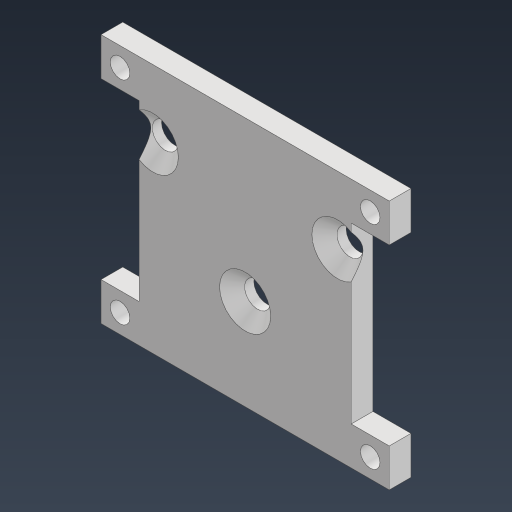
# Autodesk Inventor part: vesc_holder
Saved by Autodesk Inventor 2023 (Build 270158000, 158)
## iProperties
Created: 2026-01-23
Part Number: vesc_holder
Material: Generic
Document SubType Name: Modeling
Designer: szymo
Density: 1 g/cm^3
Appearance: Default
Author: szymo
Autodesk Inventor part; units mm, degrees
ref_plane "YZ Plane" through (0, 0, 0) normal (1, 0, 0) x (0, 1, 0)
ref_plane "XZ Plane" through (0, 0, 0) normal (0, 1, 0) x (-1, 0, 0)
ref_plane "XY Plane" through (0, 0, 0) normal (0, 0, 1) x (1, 0, 0)
sketch "Sketch1" plane through (0, 0, 0) normal (0, 0, 1) x (1, 0, 0)
  circle A0 centre (16.975, 77.075) radius 1.621 projected
  circle A1 centre (0, 60.25) radius 1.621 projected
  circle A2 centre (-16.975, 77.075) radius 1.621 projected
  line L0 (-19.5, 89.5) -> (-19.5, 43.5) projected
  line L1 (-19.5, 43.5) -> (-13.8, 43.5) projected
  line L2 (-13.8, 43.5) -> (-13.8, 49.1) projected
  arc A3 (-10.8, 52.1) -> (-13.8, 49.1) centre (-10.8, 49.1) ccw projected
  line L3 (-10.8, 52.1) -> (10.8, 52.1) projected
  arc A4 (13.8, 49.1) -> (10.8, 52.1) centre (10.8, 49.1) ccw projected
  line L4 (13.8, 49.1) -> (13.8, 43.5) projected
  line L5 (13.8, 43.5) -> (19.5, 43.5) projected
  line L6 (19.5, 43.5) -> (19.5, 89.5) projected
  line L7 (19.5, 89.5) -> (-19.5, 89.5) projected
  circle A5 centre (-17, 46.5) radius 1.25 projected
  circle A6 centre (17, 46.5) radius 1.25 projected
  circle A7 centre (17, 86.5) radius 1.25 projected
  circle A8 centre (-17, 86.5) radius 1.25 projected
  line L8 (-19.5, 89.5) -> (19.5, 89.5)
  line L9 (19.5, 89.5) -> (19.5, 43.5)
  line L10 (19.5, 43.5) -> (-19.5, 43.5)
  line L11 (-19.5, 43.5) -> (-19.5, 89.5)
  point P0 (0, 0)
  point P1 (-13.8, 43.5)
  point P2 (13.8, 43.5)
  constraints: 8 end point, 2 parallel, 1 horizontal, 1 perpendicular
extrude "Extrusion1" add sketch "Sketch1" along normal blind 4 contours A0 | A1 | A2 | L7 L6 L5 L4 A4 L3 A3 L2 L1 L0 | L2 A3 L3 A4 L4 L10 | A5 | A6 | A7 | A8
sketch "Sketch2" plane through (0, 0, 4) normal (0, 0, 1) x (1, 0, 0)
  circle A0 centre (16.975, 77.075) radius 1.621 projected
  circle A1 centre (0, 60.25) radius 1.621 projected
  circle A2 centre (-16.975, 77.075) radius 1.621 projected
  line L0 (-19.5, 89.5) -> (-19.5, 43.5) projected
  line L1 (-19.5, 43.5) -> (-13.8, 43.5) projected
  line L2 (-13.8, 43.5) -> (-13.8, 49.1) projected
  arc A3 (-10.8, 52.1) -> (-13.8, 49.1) centre (-10.8, 49.1) ccw projected
  line L3 (-10.8, 52.1) -> (10.8, 52.1) projected
  arc A4 (13.8, 49.1) -> (10.8, 52.1) centre (10.8, 49.1) ccw projected
  line L4 (13.8, 49.1) -> (13.8, 43.5) projected
  line L5 (13.8, 43.5) -> (19.5, 43.5) projected
  line L6 (19.5, 43.5) -> (19.5, 89.5) projected
  line L7 (19.5, 89.5) -> (-19.5, 89.5) projected
  circle A5 centre (-17, 46.5) radius 1.25 projected
  circle A6 centre (17, 46.5) radius 1.25 projected
  circle A7 centre (17, 86.5) radius 1.25 projected
  circle A8 centre (-17, 86.5) radius 1.25 projected
  point P0 (0, 0)
  constraints: 3 coincident
hole "Hole1" at (-16.975, 77.075, 4) at (16.975, 77.075, 4) at (0, 60.25, 4) direction (0, 0, -1) diameter 4.8 depth 5 countersink diameter 9.4 countersink angle 90 clearance for "Countersunk Flat Head Screw ISO 2009/7046" size "M4" standard "ISO"
sketch "Sketch3" plane through (0, 0, 0) normal (0, 0, -1) x (-1, 0, 0)
  line L0 (-19.5, 81.0391) -> (-19.5, 89.5) projected
  line L1 (-19.5, 89.5) -> (19.5, 89.5) projected
  line L2 (19.5, 89.5) -> (19.5, 81.0391) projected
  line L3 (19.5, 43.5) -> (-19.5, 43.5) projected
  line L4 (-19.5, 89.5) -> (19.5, 89.5) projected
  line L5 (19.5, 89.5) -> (26.5, 89.5)
  line L6 (26.5, 89.5) -> (26.5, 82.5)
  line L7 (26.5, 82.5) -> (19.5, 82.5)
  line L8 (19.5, 82.5) -> (19.5, 89.5)
  line L9 (-19.5, 89.5) -> (-26.5, 89.5)
  line L10 (-26.5, 89.5) -> (-26.5, 82.5)
  line L11 (-26.5, 82.5) -> (-19.5, 82.5)
  line L12 (-19.5, 82.5) -> (-19.5, 89.5)
  line L13 (19.5, 43.5) -> (-19.5, 43.5) projected
  line L14 (19.5, 43.5) -> (26.5, 43.5)
  line L15 (26.5, 43.5) -> (26.5, 50.5)
  line L16 (26.5, 50.5) -> (19.5, 50.5)
  line L17 (19.5, 50.5) -> (19.5, 43.5)
  line L18 (-19.5, 50.5) -> (-26.5, 50.5)
  line L19 (-26.5, 50.5) -> (-26.5, 43.5)
  line L20 (-26.5, 43.5) -> (-19.5, 43.5)
  line L21 (-19.5, 43.5) -> (-19.5, 50.5)
  arc A0 (-19.5, 73.1109) -> (-19.5, 81.0391) centre (-16.975, 77.075) ccw projected
  arc A1 (19.5, 81.0391) -> (19.5, 73.1109) centre (16.975, 77.075) ccw projected
  line L22 (19.5, 73.1109) -> (19.5, 43.5) projected
  line L23 (-19.5, 43.5) -> (-19.5, 73.1109) projected
  point P0 (0, 0)
  point P1 (-19.5, 82.5)
  point P2 (19.5, 82.5)
  dimension "d9" = 7
  dimension "d10" = 7
  dimension "d11" = 7
  dimension "d12" = 7
  dimension "d15" = 7
  dimension "d16" = 7
  dimension "d17" = 7
  dimension "d18" = 7
  dimension "d19" = 0
  constraints: 32 end point, 8 parallel, 4 horizontal, 4 perpendicular
  measures "d9" distance of L6.end L7.end
  measures "d10" distance of L5.end L6.end
  measures "d11" distance of L11.end L10.end
  measures "d12" distance of L10.end L9.end
  measures "d15" distance of L16.end L15.end
  measures "d16" distance of L15.end L14.end
  measures "d17" distance of L20.end L19.end
  measures "d18" distance of L19.end L18.end
  measures "d19" distance between parallel lines of L20 L3
extrude "Extrusion2" add sketch "Sketch3" against normal up to surface (4 mm away) contours L11 L10 L9 L0 | L21 L20 L19 L18 | L5 L6 L7 L2 | L17 L16 L15 L14
sketch "Sketch4" plane through (0, 0, 0) normal (0, 0, -1) x (-1, 0, 0)
  line L0 (26.5, 43.5) -> (-26.5, 43.5) projected
  line L1 (26.5, 43.5) -> (26.5, 50.5) projected
  line L2 (26.5, 50.5) -> (19.5, 50.5) projected
  line L3 (19.5, 82.5) -> (19.5, 50.5) projected
  line L4 (19.5, 82.5) -> (26.5, 82.5) projected
  line L5 (26.5, 82.5) -> (26.5, 89.5) projected
  line L6 (26.5, 89.5) -> (-26.5, 89.5) projected
  line L7 (-26.5, 89.5) -> (-26.5, 82.5) projected
  line L8 (-26.5, 82.5) -> (-19.5, 82.5) projected
  line L9 (-19.5, 50.5) -> (-19.5, 82.5) projected
  line L10 (-19.5, 50.5) -> (-26.5, 50.5) projected
  line L11 (-26.5, 50.5) -> (-26.5, 43.5) projected
  line L12 (26.5, 50.5) -> (19.5, 43.5)
  line L13 (19.5, 82.5) -> (19.5, 50.5) projected
  line L14 (26.5, 43.5) -> (19.5, 50.5)
  line L15 (-26.5, 50.5) -> (-26.5, 43.5) projected
  line L16 (-26.5, 50.5) -> (-19.5, 43.5)
  line L17 (-26.5, 43.5) -> (-19.5, 50.5)
  line L18 (26.5, 89.5) -> (19.5, 82.5)
  line L19 (26.5, 82.5) -> (19.5, 89.5)
  line L20 (-19.5, 50.5) -> (-19.5, 82.5) projected
  line L21 (-26.5, 89.5) -> (-19.5, 82.5)
  line L22 (-19.5, 82.5) -> (-26.5, 82.5)
  line L23 (-26.5, 82.5) -> (-19.5, 89.5)
  point P0 (0, 0)
  point P1 (19.5, 73.1109)
  point P2 (-19.5, 81.0391)
  point P3 (23, 47)
  point P4 (-23, 47)
  point P5 (-23, 86)
  point P6 (23, 86)
  constraints: 18 end point, 5 midpoint, 5 point on line, 3 perpendicular, 2 parallel, 1 horizontal
hole "Hole2" at (-23, 47, 0) at (23, 47, 0) at (23, 86, 0) at (-23, 86, 0) direction (0, 0, 1) diameter 3.6 depth 5 clearance for "Countersunk Flat Head Screw ISO 2009/7046" size "M3" standard "ISO"
body "Solid1"
